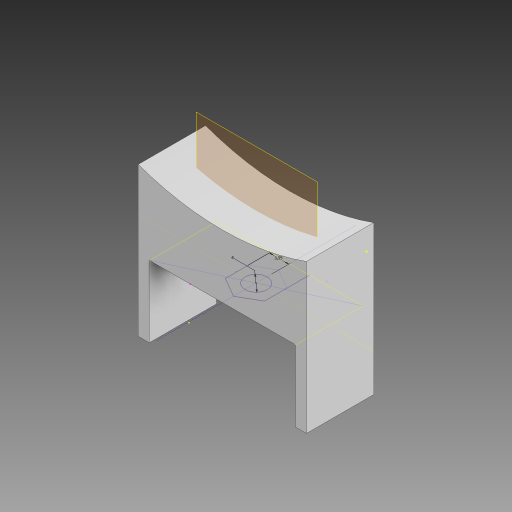
# Autodesk Inventor part: kicker1.1
Saved by Autodesk Inventor 2023 (Build 270158000, 158)
## iProperties
Created: 2025-04-11
Part Number: kicker1.1
Material: Типовые
Document SubType Name: Modeling
Designer: Ivan
Density: 1 g/cm^3
Appearance: По умолчанию
Author: Ivan
Autodesk Inventor part; units mm, degrees
ref_plane "YZ Plane" through (0, 0, 0) normal (1, 0, 0) x (0, 1, 0)
ref_plane "XZ Plane" through (0, 0, 0) normal (0, 1, 0) x (-1, 0, 0)
ref_plane "XY Plane" through (0, 0, 0) normal (0, 0, 1) x (1, 0, 0)
ref_plane "РабПлоскость2" through (19.838, 4.4675, -12.3) normal (0, 0, 1) x (1, 0, 0)
ref_plane "РабПлоскость1" through (-13.412, 18.3334, -19.05) normal (0, 0, 1) x (1, 0, 0)
sketch "Эскиз1" plane through (19.838, 4.4675, -12.3) normal (0, 0, 1) x (1, 0, 0)
  line L0 (-17.838, -7.8158) -> (-21.838, -7.8158) projected
  line L1 (-21.838, -12.9158) -> (-17.838, -12.9158) projected
  line L2 (-15.838, -12.5585) -> (-15.838, -8.173) projected
  line L3 (-23.838, -12.5585) -> (-23.838, -8.173) projected
  line L4 (-15.688, -12.9158) -> (-23.988, -12.9158)
  line L5 (-23.988, -12.9158) -> (-23.988, -7.5158)
  line L6 (-23.988, -7.5158) -> (-15.688, -7.5158)
  line L7 (-15.688, -7.5158) -> (-15.688, -12.9158)
  line L8 (-15.688, -12.9158) -> (-23.988, -7.5158) construction
  line L9 (-19.838, -4.4675) -> (-19.838, -10.2158) construction
  line L10 (-15.388, -12.9158) -> (-24.288, -12.9158)
  line L11 (-6.75, -10.8528) -> (-33.25, -10.8528) projected
  line L12 (-33.25, -10.8528) -> (-6.75, -10.8528) projected
  line L13 (-33.25, -10.8528) -> (-6.75, -10.8528) construction
  line L14 (-24.938, -14.0158) -> (-14.738, -14.0158) projected
  line L15 (-15.388, -12.9158) -> (-24.288, -12.9158)
  line L16 (-19.838, -14.0158) -> (-19.838, -12.9158) construction
  line L17 (-13.838, -13.4658) -> (-25.838, -13.4658) construction
  line L18 (-25.838, -13.4658) -> (-25.838, -3.5158)
  line L19 (-25.838, -3.5158) -> (-13.838, -3.5158)
  line L20 (-13.838, -3.5158) -> (-13.838, -13.4658)
  line L21 (-6.75, -10.8528) -> (-33.25, -10.8528)
  line L22 (-33.25, -10.8528) -> (-33.25, -3.5158) construction
  line L23 (-33.25, -3.5158) -> (-6.75, -3.5158)
  line L24 (-6.75, -3.5158) -> (-6.75, -10.8528) construction
  line L25 (-6.75, -3.5158) -> (-6.75, -1.5158) construction
  line L26 (-33.25, -3.5158) -> (-33.25, -1.5158) construction
  arc A0 (-33.25, -1.5158) -> (-6.75, -1.5158) centre (-20, 41.3683) ccw
  line L27 (-25.838, -13.4658) -> (-13.838, -13.4658) construction
  line L28 (-13.838, -13.4658) -> (-25.838, -13.4658)
  line L29 (-4.75, -0.8459) -> (-4.75, -27.8528)
  line L30 (-35.25, -0.8459) -> (-35.25, -27.8528)
  arc A1 (-35.25, -0.8459) -> (-33.25, -1.5158) centre (-20, 41.3683) ccw
  arc A2 (-6.75, -1.5158) -> (-4.75, -0.8459) centre (-20, 41.3683) ccw
  line L31 (-33.25, -14.9158) -> (-33.25, -27.8528)
  line L32 (-33.25, -27.8528) -> (-35.25, -27.8528)
  line L33 (-6.75, -14.9158) -> (-6.75, -27.8528)
  line L34 (-6.75, -27.8528) -> (-4.75, -27.8528)
  line L35 (-33.25, -14.9158) -> (-6.75, -14.9158)
  point P0 (-19.838, -13.4658)
  point P1 (-19.838, -3.5158)
  point P2 (-25.838, -10.8528)
  point P3 (-13.838, -10.8528)
  point P4 (-20.162, -3.5158)
  point P5 (-15.688, -10.8528)
  point P6 (-23.988, -10.8528)
  point P7 (-20.162, -3.5158)
  point P8 (-17.838, -12.9158)
  dimension "d0" = 8.3
  dimension "d1" = 5.4
  dimension "d2" = 12
  dimension "d3" = 4
  dimension "d4" = 2
  dimension "d10" = 0
  dimension "d11" = 0.55
  dimension "d26" = 2
  dimension "d27" = 2
  dimension "d30" = 17
  dimension "d33" = 2
  constraints: 56 end point, 9 point on circle, 8 horizontal, 8 vertical, 7 equal length, 7 midpoint, 5 perpendicular, 4 point on line, 3 centre point, 2 coincident, 2 concentric, 2 parallel, 6 other
  measures "d0" distance between parallel lines of L5 L7
  measures "d1" distance between parallel lines of L4 L6
  measures "d2" distance between parallel lines of L20 L18
  measures "d3" distance from line of L6 point (-19.838, -3.516)
  measures "d4" distance of L22.end L26.end
  measures "d10" distance of L27.end L28.start
  measures "d11" distance between parallel lines of L4 L28
  measures "d26" distance between parallel lines of L24 L29
  measures "d27" distance between parallel lines of L30 L22
  measures "d30" distance between parallel lines of L34 L21
  measures "d33" distance between parallel lines of L4 L35
extrude "Выдавливание1" add sketch "Эскиз1" along normal mid plane 12.2 contours L4 L5 L11 L7 L1 | L1 L4 L7 L11 L20 L28 L18 L5 | L11 L18 L19 L20 L7 L6 L5 | L5 L6 L7 L11 | A0 A2 L29 L34 L33 L35 L31 L32 L30 A1
sketch "Эскиз3" plane through (-6, -10.4482, -6.2) normal (0, -1, 0) x (1, 0, 0)
  circle A0 centre (5.838, -6.1) radius 2
  line L0 (19.088, -12.2) -> (19.088, 0) projected
  line L1 (-7.412, -12.2) -> (-7.412, 0) projected
  line L2 (-7.412, 0) -> (19.088, -12.2) construction
  line L3 (5.838, 12.0241) -> (5.838, -24.2241) construction
  line L4 (-15.512, -6.1) -> (27.188, -6.1) construction
  line L5 (2.288, -4.0504) -> (5.838, -2.0008)
  line L6 (5.838, -2.0008) -> (9.388, -4.0504)
  line L7 (9.388, -4.0504) -> (9.388, -8.1496)
  line L8 (9.388, -8.1496) -> (5.838, -10.1992) construction
  line L9 (5.838, -10.1992) -> (2.288, -8.1496) construction
  line L10 (2.288, -8.1496) -> (2.288, -4.0504)
  line L11 (2.288, -8.1496) -> (2.288, -12.2488)
  line L12 (9.388, -8.1496) -> (9.388, -12.2)
  line L13 (19.088, -12.2) -> (-7.412, -12.2) projected
  point P0 (6, 6.2)
  point P1 (0, 0)
  point P2 (12, -12.8)
  point P3 (5.838, -6.1)
  point P4 (5.838, -6.1)
  point P5 (2.288, -6.1)
  point P6 (2.288, -12.2)
  dimension "d12" = 4
  dimension "d34" = 3.55
  constraints: 20 end point, 5 midpoint, 3 vertical, 2 coincident, 2 point on line, 1 centre point, 13 other
  measures "d12" diameter of A0
  measures "d34" distance between parallel lines of L10 L3
extrude "Выдавливание8" cut sketch "Эскиз3" against normal blind 5.3 contours A0 | L5 L6 L7 L12 L13 L11 L10
extrude "Выдавливание9" add sketch "Эскиз3" against normal blind 2
extrude "Выдавливание10" cut sketch "Эскиз3" against normal blind 7 contours A0
equation "\"d27\" = d26"
